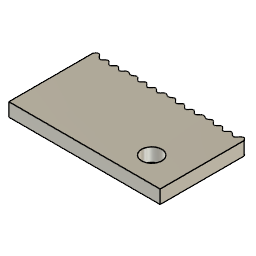
fixture-tiny-segment-storm (Autodesk Fusion 360 design; units mm, degrees)
part number: 2026-04-07-17-31-53-805
Autodesk Fusion 360 part; units mm, degrees
sketch "sketch_dense_outline" plane through (0, 0, 0) normal (0, 0, 1) x (1, 0, 0)
  spline S0 degree 5 poles (0, 50) (0.1252, 50.2322) (0.374, 50.6565) (0.7426, 51.1728) (1.2247, 51.6208) (1.8119, 51.7906) (2.3847, 51.6025) (2.9445, 51.1198) (3.4942, 50.4508) (4.0378, 49.7503) (4.5795, 49.1813) (5.1235, 48.8824) (5.6728, 48.9345) (6.2286, 49.3244) (6.79, 49.9179) (7.3544, 50.5193) (7.9185, 50.9269) (8.4792, 50.988) (9.0346, 50.6575) (9.5841, 50.047) (10.1288, 49.3559) (10.6704, 48.8102) (11.2112, 48.5963) (11.7534, 48.8004) (12.2989, 49.3382) (12.8492, 50.0165) (13.4046, 50.6025) (13.9652, 50.8919) (14.5295, 50.7732) (15.0953, 50.3067) (15.6595, 49.6746) (16.2193, 49.1069) (16.7729, 48.8128) (17.3203, 48.916) (17.8641, 49.3732) (18.4086, 50.0193) (18.959, 50.6398) (19.5197, 51.0356) (20.094, 51.0848) (20.6822, 50.824) (21.2821, 50.4127) (21.8898, 50.0532) (22.5005, 49.9234) (23.1091, 50.1055) (23.7111, 50.5156) (24.3025, 50.9735) (24.8811, 51.2737) (25.446, 51.2525) (25.9987, 50.8659) (26.5429, 50.2331) (27.0834, 49.5549) (27.6253, 49.053) (28.1724, 48.902) (28.7269, 49.1612) (29.2879, 49.7167) (29.8527, 50.359) (30.4177, 50.8514) (30.9794, 51.0004) (31.5353, 50.7284) (32.085, 50.1369) (32.6296, 49.4302) (33.1708, 48.8485) (33.7112, 48.5957) (34.2531, 48.7726) (34.7986, 49.3002) (35.3488, 49.9838) (35.9045, 50.5845) (36.4652, 50.8907) (37.0297, 50.7841) (37.5955, 50.3225) (38.1596, 49.6886) (38.7194, 49.1147) (39.2729, 48.8135) (39.8203, 48.9114) (40.364, 49.3663) (40.9086, 50.0132) (41.4589, 50.6362) (42.0197, 51.0351) (42.594, 51.0865) (43.1822, 50.8265) (43.7821, 50.415) (44.3898, 50.0543) (45.0005, 49.9233) (45.6091, 50.1046) (46.211, 50.5145) (46.8025, 50.9726) (47.3811, 51.2733) (47.946, 51.2526) (48.4987, 50.8664) (49.0429, 50.2336) (49.5835, 49.5553) (50.1253, 49.0532) (50.6724, 48.902) (51.2269, 49.161) (51.7879, 49.7165) (52.3527, 50.3588) (52.9177, 50.8513) (53.4794, 51.0004) (54.0353, 50.7285) (54.585, 50.137) (55.1296, 49.4303) (55.6708, 48.8486) (56.2112, 48.5957) (56.7531, 48.7725) (57.2986, 49.3001) (57.8488, 49.9836) (58.4045, 50.5844) (58.9652, 50.8907) (59.5297, 50.7842) (60.0955, 50.3227) (60.6596, 49.6888) (61.2194, 49.1149) (61.7729, 48.8135) (62.3203, 48.9112) (62.8641, 49.3659) (63.4086, 50.0127) (63.959, 50.6357) (64.5197, 51.0349) (65.094, 51.0869) (65.6822, 50.8274) (66.2821, 50.4161) (66.8898, 50.0552) (67.5005, 49.9234) (68.1092, 50.1035) (68.7111, 50.5123) (69.3026, 50.97) (69.8811, 51.2715) (70.446, 51.253) (70.9987, 50.8698) (71.5428, 50.2396) (72.0833, 49.5622) (72.6252, 49.0581) (73.1724, 48.9019) (73.727, 49.154) (74.2881, 49.7032) (74.853, 50.3431) (75.4179, 50.8397) (75.9794, 51.0002) (76.535, 50.7446) (77.0845, 50.1683) (77.6289, 49.4683) (78.1703, 48.8786) (78.7111, 48.601) (79.2536, 48.7404) (79.7997, 49.2315) (80.3502, 49.8967) (80.9056, 50.5118) (81.4655, 50.8713) (82.0286, 50.8489) (82.593, 50.4724) (83.1564, 49.8846) (83.7166, 49.2821) (84.2721, 48.8617) (84.8227, 48.7657) (85.3697, 49.0193) (85.9162, 49.5497) (86.4658, 50.2248) (87.0223, 50.8854) (87.5892, 51.3783) (88.1689, 51.5946) (88.7629, 51.4708) (89.2501, 51.0739) (89.6224, 50.604) (89.8736, 50.2141) (90, 50) knots 0 0 0 0 0 0 0.00625 0.0125 0.01875 0.025 0.03125 0.0375 0.04375 0.05 0.05625 0.0625 0.06875 0.075 0.08125 0.0875 0.09375 0.1 0.10625 0.1125 0.11875 0.125 0.13125 0.1375 0.14375 0.15 0.15625 0.1625 0.16875 0.175 0.18125 0.1875 0.19375 0.2 0.20625 0.2125 0.21875 0.225 0.23125 0.2375 0.24375 0.25 0.25625 0.2625 0.26875 0.275 0.28125 0.2875 0.29375 0.3 0.30625 0.3125 0.31875 0.325 0.33125 0.3375 0.34375 0.35 0.35625 0.3625 0.36875 0.375 0.38125 0.3875 0.39375 0.4 0.40625 0.4125 0.41875 0.425 0.43125 0.4375 0.44375 0.45 0.45625 0.4625 0.46875 0.475 0.48125 0.4875 0.49375 0.5 0.50625 0.5125 0.51875 0.525 0.53125 0.5375 0.54375 0.55 0.55625 0.5625 0.56875 0.575 0.58125 0.5875 0.59375 0.6 0.60625 0.6125 0.61875 0.625 0.63125 0.6375 0.64375 0.65 0.65625 0.6625 0.66875 0.675 0.68125 0.6875 0.69375 0.7 0.70625 0.7125 0.71875 0.725 0.73125 0.7375 0.74375 0.75 0.75625 0.7625 0.76875 0.775 0.78125 0.7875 0.79375 0.8 0.80625 0.8125 0.81875 0.825 0.83125 0.8375 0.84375 0.85 0.85625 0.8625 0.86875 0.875 0.88125 0.8875 0.89375 0.9 0.90625 0.9125 0.91875 0.925 0.93125 0.9375 0.94375 0.95 0.95625 0.9625 0.96875 0.975 0.98125 0.9875 0.99375 1 1 1 1 1 1
  line L0 (0, 0) -> (0, 50)
  line L1 (90, 50) -> (90, 0)
  line L2 (90, 0) -> (0, 0)
  point P0 (2.8125, 51.2)
  point P1 (5.625, 49)
  point P2 (8.4375, 50.9)
  point P3 (11.25, 48.7)
  point P4 (14.0625, 50.8)
  point P5 (16.875, 48.9)
  point P6 (19.6875, 51)
  point P7 (22.5, 50)
  point P8 (25.3125, 51.2)
  point P9 (28.125, 49)
  point P10 (30.9375, 50.9)
  point P11 (33.75, 48.7)
  point P12 (36.5625, 50.8)
  point P13 (39.375, 48.9)
  point P14 (42.1875, 51)
  point P15 (45, 50)
  point P16 (47.8125, 51.2)
  point P17 (50.625, 49)
  point P18 (53.4375, 50.9)
  point P19 (56.25, 48.7)
  point P20 (59.0625, 50.8)
  point P21 (61.875, 48.9)
  point P22 (64.6875, 51)
  point P23 (67.5, 50)
  point P24 (70.3125, 51.2)
  point P25 (73.125, 49)
  point P26 (75.9375, 50.9)
  point P27 (78.75, 48.7)
  point P28 (81.5625, 50.8)
  point P29 (84.375, 48.9)
  point P30 (87.1875, 51)
extrude "Extrude1" add sketch "sketch_dense_outline" along normal blind 8
sketch "sketch_bore_reference" plane through (0, 0, 8) normal (0, 0, 1) x (1, 0, 0)
  line L0 (90, 0) -> (90, 50)
  spline S0 degree 5 poles (90, 50) (89.8736, 50.2141) (89.6224, 50.604) (89.2501, 51.0739) (88.7629, 51.4708) (88.1689, 51.5946) (87.5892, 51.3783) (87.0223, 50.8854) (86.4658, 50.2248) (85.9162, 49.5497) (85.3697, 49.0193) (84.8227, 48.7657) (84.2721, 48.8617) (83.7166, 49.2821) (83.1564, 49.8846) (82.593, 50.4724) (82.0286, 50.8489) (81.4655, 50.8713) (80.9056, 50.5118) (80.3502, 49.8967) (79.7997, 49.2315) (79.2536, 48.7404) (78.7111, 48.601) (78.1703, 48.8786) (77.6289, 49.4683) (77.0845, 50.1683) (76.535, 50.7446) (75.9794, 51.0002) (75.4179, 50.8397) (74.853, 50.3431) (74.2881, 49.7032) (73.727, 49.154) (73.1724, 48.9019) (72.6252, 49.0581) (72.0833, 49.5622) (71.5428, 50.2396) (70.9987, 50.8698) (70.446, 51.253) (69.8811, 51.2715) (69.3026, 50.97) (68.7111, 50.5123) (68.1092, 50.1035) (67.5005, 49.9234) (66.8898, 50.0552) (66.2821, 50.4161) (65.6822, 50.8274) (65.094, 51.0869) (64.5197, 51.0349) (63.959, 50.6357) (63.4086, 50.0127) (62.8641, 49.3659) (62.3203, 48.9112) (61.7729, 48.8135) (61.2194, 49.1149) (60.6596, 49.6888) (60.0955, 50.3227) (59.5297, 50.7842) (58.9652, 50.8907) (58.4045, 50.5844) (57.8488, 49.9836) (57.2986, 49.3001) (56.7531, 48.7725) (56.2112, 48.5957) (55.6708, 48.8486) (55.1296, 49.4303) (54.585, 50.137) (54.0353, 50.7285) (53.4794, 51.0004) (52.9177, 50.8513) (52.3527, 50.3588) (51.7879, 49.7165) (51.2269, 49.161) (50.6724, 48.902) (50.1253, 49.0532) (49.5835, 49.5553) (49.0429, 50.2336) (48.4987, 50.8664) (47.946, 51.2526) (47.3811, 51.2733) (46.8025, 50.9726) (46.211, 50.5145) (45.6091, 50.1046) (45.0005, 49.9233) (44.3898, 50.0543) (43.7821, 50.415) (43.1822, 50.8265) (42.594, 51.0865) (42.0197, 51.0351) (41.4589, 50.6362) (40.9086, 50.0132) (40.364, 49.3663) (39.8203, 48.9114) (39.2729, 48.8135) (38.7194, 49.1147) (38.1596, 49.6886) (37.5955, 50.3225) (37.0297, 50.7841) (36.4652, 50.8907) (35.9045, 50.5845) (35.3488, 49.9838) (34.7986, 49.3002) (34.2531, 48.7726) (33.7112, 48.5957) (33.1708, 48.8485) (32.6296, 49.4302) (32.085, 50.1369) (31.5353, 50.7284) (30.9794, 51.0004) (30.4177, 50.8514) (29.8527, 50.359) (29.2879, 49.7167) (28.7269, 49.1612) (28.1724, 48.902) (27.6253, 49.053) (27.0834, 49.5549) (26.5429, 50.2331) (25.9987, 50.8659) (25.446, 51.2525) (24.8811, 51.2737) (24.3025, 50.9735) (23.7111, 50.5156) (23.1091, 50.1055) (22.5005, 49.9234) (21.8898, 50.0532) (21.2821, 50.4127) (20.6822, 50.824) (20.094, 51.0848) (19.5197, 51.0356) (18.959, 50.6398) (18.4086, 50.0193) (17.8641, 49.3732) (17.3203, 48.916) (16.7729, 48.8128) (16.2193, 49.1069) (15.6595, 49.6746) (15.0953, 50.3067) (14.5295, 50.7732) (13.9652, 50.8919) (13.4046, 50.6025) (12.8492, 50.0165) (12.2989, 49.3382) (11.7534, 48.8004) (11.2112, 48.5963) (10.6704, 48.8102) (10.1288, 49.3559) (9.5841, 50.047) (9.0346, 50.6575) (8.4792, 50.988) (7.9185, 50.9269) (7.3544, 50.5193) (6.79, 49.9179) (6.2286, 49.3244) (5.6728, 48.9345) (5.1235, 48.8824) (4.5795, 49.1813) (4.0378, 49.7503) (3.4942, 50.4508) (2.9445, 51.1198) (2.3847, 51.6025) (1.8119, 51.7906) (1.2247, 51.6208) (0.7426, 51.1728) (0.374, 50.6565) (0.1252, 50.2322) (0, 50) knots -1 -1 -1 -1 -1 -1 -0.99375 -0.9875 -0.98125 -0.975 -0.96875 -0.9625 -0.95625 -0.95 -0.94375 -0.9375 -0.93125 -0.925 -0.91875 -0.9125 -0.90625 -0.9 -0.89375 -0.8875 -0.88125 -0.875 -0.86875 -0.8625 -0.85625 -0.85 -0.84375 -0.8375 -0.83125 -0.825 -0.81875 -0.8125 -0.80625 -0.8 -0.79375 -0.7875 -0.78125 -0.775 -0.76875 -0.7625 -0.75625 -0.75 -0.74375 -0.7375 -0.73125 -0.725 -0.71875 -0.7125 -0.70625 -0.7 -0.69375 -0.6875 -0.68125 -0.675 -0.66875 -0.6625 -0.65625 -0.65 -0.64375 -0.6375 -0.63125 -0.625 -0.61875 -0.6125 -0.60625 -0.6 -0.59375 -0.5875 -0.58125 -0.575 -0.56875 -0.5625 -0.55625 -0.55 -0.54375 -0.5375 -0.53125 -0.525 -0.51875 -0.5125 -0.50625 -0.5 -0.49375 -0.4875 -0.48125 -0.475 -0.46875 -0.4625 -0.45625 -0.45 -0.44375 -0.4375 -0.43125 -0.425 -0.41875 -0.4125 -0.40625 -0.4 -0.39375 -0.3875 -0.38125 -0.375 -0.36875 -0.3625 -0.35625 -0.35 -0.34375 -0.3375 -0.33125 -0.325 -0.31875 -0.3125 -0.30625 -0.3 -0.29375 -0.2875 -0.28125 -0.275 -0.26875 -0.2625 -0.25625 -0.25 -0.24375 -0.2375 -0.23125 -0.225 -0.21875 -0.2125 -0.20625 -0.2 -0.19375 -0.1875 -0.18125 -0.175 -0.16875 -0.1625 -0.15625 -0.15 -0.14375 -0.1375 -0.13125 -0.125 -0.11875 -0.1125 -0.10625 -0.1 -0.09375 -0.0875 -0.08125 -0.075 -0.06875 -0.0625 -0.05625 -0.05 -0.04375 -0.0375 -0.03125 -0.025 -0.01875 -0.0125 -0.00625 0 0 0 0 0 0
  line L1 (0, 50) -> (0, 0)
  line L2 (0, 0) -> (90, 0)
  circle A0 centre (70, 15) radius 6
extrude "bore_reference_hole" cut sketch "sketch_bore_reference" against normal blind 8 contours A0
equation "d3 = -( 8 mm )"
named bodies: "storm_fixture_body"
